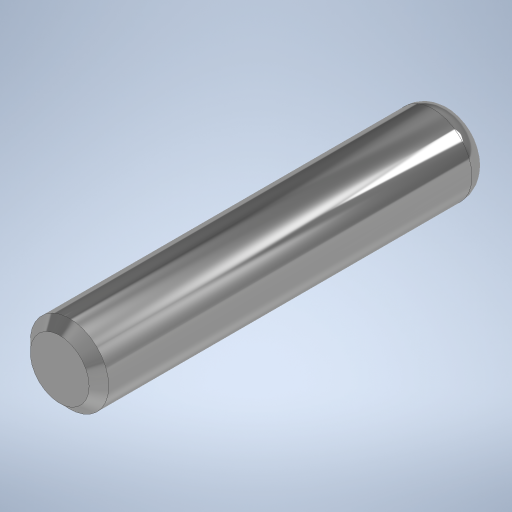
# Autodesk Inventor part: DOWEL,M4X20
Saved by Autodesk Inventor 2024.2 (Build 282272000, 272)
## iProperties
Created: 2024-02-17
Part Number: DOWEL,M4X20
Material: Steel
Document SubType Name: Modeling
Designer: Phil.Brown
Density: 7.85 g/cm^3
Appearance: No Tint
Author: Phil.Brown
Autodesk Inventor part; units mm, degrees
ref_plane "YZ Plane" through (0, 0, 0) normal (1, 0, 0) x (0, 1, 0)
ref_plane "XZ Plane" through (0, 0, 0) normal (0, 1, 0) x (-1, 0, 0)
ref_plane "XY Plane" through (0, 0, 0) normal (0, 0, 1) x (1, 0, 0)
sketch "Sketch1" plane through (0, 0, 0) normal (0, 0, 1) x (1, 0, 0)
  circle A0 centre (0, 0) radius 2
  dimension "d0" = 4
  constraints: 1 centre point, 1 coincident
  measures "d0" diameter of A0
extrude "Extrusion1" add sketch "Sketch1" along normal mid plane 20
fillet "Fillet1" radius 1 1 edges at (-2, 0, -10)
chamfer "Chamfer1" distance 0.5 angle 45 1 edges at (-2, 0, 10)
body "Solid1"
